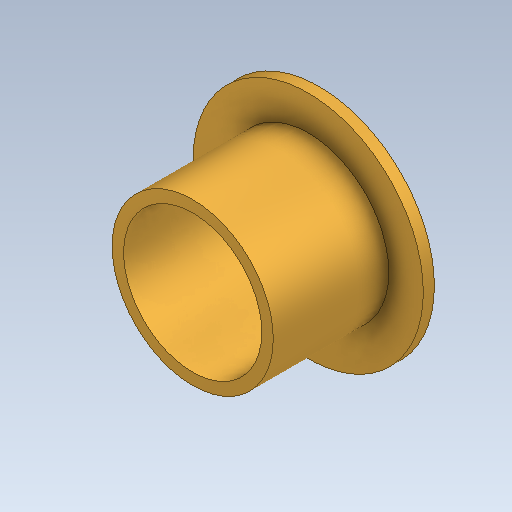
# Autodesk Inventor part: ドライメッシュw5.5f6-7a
Saved by Autodesk Inventor 2020 (Build 240168000, 168)
## iProperties
Created: 2020-04-10
Part Number: ドライメッシュw5.5f6-7a
Material: 真鍮、ソフト イエロー
Document SubType Name: Modeling
Designer: happy
Mass: 0.63849 g
Surface Area: 3.29679 cm^2
Volume: 0.0753825 cm^3
Density: 8.47 g/cm^3
Appearance: 真鍮 - サテン
Author: happy
Autodesk Inventor part; units mm, degrees
ref_plane "YZ Plane" through (0, 0, 0) normal (1, 0, 0) x (0, 1, 0)
ref_plane "XZ Plane" through (0, 0, 0) normal (0, 1, 0) x (-1, 0, 0)
ref_plane "XY Plane" through (0, 0, 0) normal (0, 0, 1) x (1, 0, 0)
sketch "スケッチ1" plane through (0, 0, 0) normal (0, 0, 1) x (1, 0, 0)
  circle A0 centre (0, 0) radius 3
  circle A1 centre (0, 0) radius 3.5
  dimension "d0" = 6
  dimension "d1" = 7
  constraints: 2 centre point, 2 coincident
  measures "d0" diameter of A0
  measures "d1" diameter of A1
extrude "押し出し1" add sketch "スケッチ1" along normal blind 5.5
sketch "スケッチ2" plane through (0, 0, 0) normal (0, 0, -1) x (-1, 0, 0)
  circle A0 centre (0, 0) radius 3.5 projected
  circle A1 centre (0, 0) radius 5
  dimension "d6" = 10
  constraints: 1 centre point, 1 coincident
  measures "d6" diameter of A1
extrude "押し出し2" add sketch "スケッチ2" against normal blind 0.48
